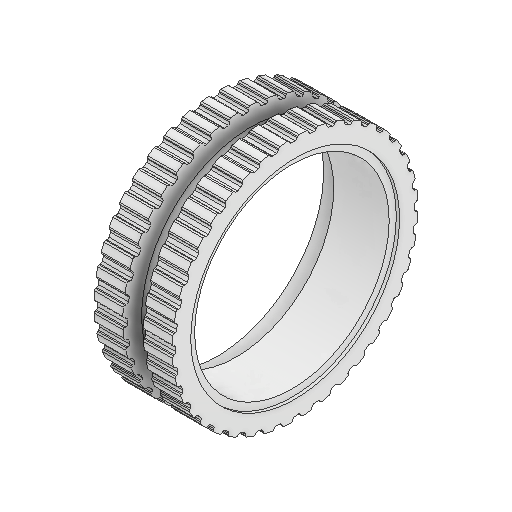
# Autodesk Inventor part: hoverboardPulleyAdapter
Saved by Autodesk Inventor 2025 (Build 290162000, 162)
## iProperties
Created: 2024-06-22
Part Number: hoverboardPulleyAdapter
Material: ABS Plastic
Document SubType Name: Modeling
Designer: derm
Density: 1.06 g/cm^3
Appearance: Smooth - White
Mass: 267.013 g
Surface Area: 496.078 cm^2
Volume: 251.899 cm^3
Author: derm
Autodesk Inventor part; units mm, degrees
ref_plane "YZ Plane" through (0, 0, 0) normal (1, 0, 0) x (0, 1, 0)
ref_plane "XZ Plane" through (0, 0, 0) normal (0, 1, 0) x (-1, 0, 0)
ref_plane "XY Plane" through (0, 0, 0) normal (0, 0, 1) x (1, 0, 0)
sketch "Sketch1" plane through (0, 0, 0) normal (1, 0, 0) x (0, 1, 0)
  circle A0 centre (0, 0) radius 63.119
  circle A1 centre (0, 0) radius 72.4459 projected
  arc A2 (-69.867, -16.1918) -> (-68.6025, -20.911) centre (0, 0) ccw projected
  arc A3 (-69.3853, -15.0825) -> (-69.867, -16.1918) centre (-68.8773, -15.9624) ccw projected
  line L0 (-69.3853, -15.0825) -> (-68.7891, -14.7383) projected
  arc A4 (-68.7891, -14.7383) -> (-68.0995, -13.2595) centre (-69.5003, -13.5065) ccw projected
  line L1 (-68.0995, -13.2595) -> (-68.5276, -10.8316) projected
  arc A5 (-68.5276, -10.8316) -> (-69.6814, -9.6778) centre (-69.9284, -11.0786) ccw projected
  line L2 (-69.6814, -9.6778) -> (-70.3594, -9.5582) projected
  arc A6 (-71.1915, -8.6806) -> (-70.3594, -9.5582) centre (-70.1829, -8.5577) ccw projected
  arc A7 (-71.6173, -3.8135) -> (-71.1915, -8.6806) centre (0, 0) ccw projected
  arc A8 (-70.9502, -2.8048) -> (-71.6173, -3.8135) centre (-70.6027, -3.7595) ccw projected
  line L3 (-70.9502, -2.8048) -> (-70.3033, -2.5693) projected
  arc A9 (-70.3033, -2.5693) -> (-69.3674, -1.2327) centre (-70.7898, -1.2327) ccw projected
  line L4 (-69.3674, -1.2327) -> (-69.3674, 1.2327) projected
  arc A10 (-69.3674, 1.2327) -> (-70.3033, 2.5693) centre (-70.7898, 1.2327) ccw projected
  line L5 (-70.3033, 2.5693) -> (-70.9502, 2.8048) projected
  arc A11 (-71.6173, 3.8135) -> (-70.9502, 2.8048) centre (-70.6027, 3.7595) ccw projected
  arc A12 (-71.1915, 8.6806) -> (-71.6173, 3.8135) centre (0, 0) ccw projected
  arc A13 (-70.3594, 9.5582) -> (-71.1915, 8.6806) centre (-70.1829, 8.5577) ccw projected
  line L6 (-70.3594, 9.5582) -> (-69.6814, 9.6778) projected
  arc A14 (-69.6814, 9.6778) -> (-68.5276, 10.8316) centre (-69.9284, 11.0786) ccw projected
  line L7 (-68.5276, 10.8316) -> (-68.0995, 13.2595) projected
  arc A15 (-68.0995, 13.2595) -> (-68.7891, 14.7383) centre (-69.5003, 13.5065) ccw projected
  line L8 (-68.7891, 14.7383) -> (-69.3853, 15.0825) projected
  arc A16 (-69.867, 16.1918) -> (-69.3853, 15.0825) centre (-68.8773, 15.9624) ccw projected
  arc A17 (-68.6025, 20.911) -> (-69.867, 16.1918) centre (0, 0) ccw projected
  arc A18 (-67.6307, 21.6308) -> (-68.6025, 20.911) centre (-67.6307, 20.6148) ccw projected
  line L9 (-67.6307, 21.6308) -> (-66.9423, 21.6308) projected
  arc A19 (-66.9423, 21.6308) -> (-65.6056, 22.5667) centre (-66.9423, 23.0532) ccw projected
  line L10 (-65.6056, 22.5667) -> (-64.7624, 24.8834) projected
  arc A20 (-64.7624, 24.8834) -> (-65.1847, 26.4595) centre (-66.099, 25.3699) ccw projected
  line L11 (-65.1847, 26.4595) -> (-65.7121, 26.902) projected
  arc A21 (-65.9939, 28.0781) -> (-65.7121, 26.902) centre (-65.059, 27.6803) ccw projected
  arc A22 (-63.9291, 32.506) -> (-65.9939, 28.0781) centre (0, 0) ccw projected
  arc A23 (-62.8471, 33.0461) -> (-63.9291, 32.506) centre (-63.0235, 32.0455) ccw projected
  line L12 (-62.8471, 33.0461) -> (-62.1691, 32.9266) projected
  arc A24 (-62.1691, 32.9266) -> (-60.6903, 33.6162) centre (-61.9221, 34.3274) ccw projected
  line L13 (-60.6903, 33.6162) -> (-59.4576, 35.7512) projected
  arc A25 (-59.4576, 35.7512) -> (-59.5998, 37.3767) centre (-60.6894, 36.4624) ccw projected
  line L14 (-59.5998, 37.3767) -> (-60.0423, 37.9041) projected
  arc A26 (-60.1156, 39.1112) -> (-60.0423, 37.9041) centre (-59.264, 38.5572) ccw projected
  arc A27 (-57.3133, 43.1134) -> (-60.1156, 39.1112) centre (0, 0) ccw projected
  arc A28 (-56.1539, 43.4573) -> (-57.3133, 43.1134) centre (-56.5014, 42.5026) ccw projected
  line L15 (-56.1539, 43.4573) -> (-55.507, 43.2219) projected
  arc A29 (-55.507, 43.2219) -> (-53.9309, 43.6442) centre (-55.0205, 44.5585) ccw projected
  line L16 (-53.9309, 43.6442) -> (-52.3462, 45.5328) projected
  arc A30 (-52.3462, 45.5328) -> (-52.2039, 47.1583) centre (-53.4358, 46.4471) ccw projected
  line L17 (-52.2039, 47.1583) -> (-52.5481, 47.7545) projected
  arc A31 (-52.4107, 48.956) -> (-52.5481, 47.7545) centre (-51.6683, 48.2625) ccw projected
  arc A32 (-48.956, 52.4107) -> (-52.4107, 48.956) centre (0, 0) ccw projected
  arc A33 (-47.7545, 52.5481) -> (-48.956, 52.4107) centre (-48.2625, 51.6683) ccw projected
  line L18 (-47.7545, 52.5481) -> (-47.1583, 52.2039) projected
  arc A34 (-47.1583, 52.2039) -> (-45.5328, 52.3462) centre (-46.4471, 53.4358) ccw projected
  line L19 (-45.5328, 52.3462) -> (-43.6442, 53.9309) projected
  arc A35 (-43.6442, 53.9309) -> (-43.2219, 55.507) centre (-44.5585, 55.0205) ccw projected
  line L20 (-43.2219, 55.507) -> (-43.4573, 56.1539) projected
  arc A36 (-43.1134, 57.3133) -> (-43.4573, 56.1539) centre (-42.5026, 56.5014) ccw projected
  arc A37 (-39.1112, 60.1156) -> (-43.1134, 57.3133) centre (0, 0) ccw projected
  arc A38 (-37.9041, 60.0423) -> (-39.1112, 60.1156) centre (-38.5572, 59.264) ccw projected
  line L21 (-37.9041, 60.0423) -> (-37.3767, 59.5998) projected
  arc A39 (-37.3767, 59.5998) -> (-35.7512, 59.4576) centre (-36.4624, 60.6894) ccw projected
  line L22 (-35.7512, 59.4576) -> (-33.6162, 60.6903) projected
  arc A40 (-33.6162, 60.6903) -> (-32.9266, 62.1691) centre (-34.3274, 61.9221) ccw projected
  line L23 (-32.9266, 62.1691) -> (-33.0461, 62.8471) projected
  arc A41 (-32.506, 63.9291) -> (-33.0461, 62.8471) centre (-32.0455, 63.0235) ccw projected
  arc A42 (-28.0781, 65.9939) -> (-32.506, 63.9291) centre (0, 0) ccw projected
  arc A43 (-26.902, 65.7121) -> (-28.0781, 65.9939) centre (-27.6803, 65.059) ccw projected
  line L24 (-26.902, 65.7121) -> (-26.4595, 65.1847) projected
  arc A44 (-26.4595, 65.1847) -> (-24.8834, 64.7624) centre (-25.3699, 66.099) ccw projected
  line L25 (-24.8834, 64.7624) -> (-22.5667, 65.6056) projected
  arc A45 (-22.5667, 65.6056) -> (-21.6308, 66.9423) centre (-23.0532, 66.9423) ccw projected
  line L26 (-21.6308, 66.9423) -> (-21.6308, 67.6307) projected
  arc A46 (-20.911, 68.6025) -> (-21.6308, 67.6307) centre (-20.6148, 67.6307) ccw projected
  arc A47 (-16.1918, 69.867) -> (-20.911, 68.6025) centre (0, 0) ccw projected
  arc A48 (-15.0825, 69.3853) -> (-16.1918, 69.867) centre (-15.9624, 68.8773) ccw projected
  line L27 (-15.0825, 69.3853) -> (-14.7383, 68.7891) projected
  arc A49 (-14.7383, 68.7891) -> (-13.2595, 68.0995) centre (-13.5065, 69.5003) ccw projected
  line L28 (-13.2595, 68.0995) -> (-10.8316, 68.5276) projected
  arc A50 (-10.8316, 68.5276) -> (-9.6778, 69.6814) centre (-11.0786, 69.9284) ccw projected
  line L29 (-9.6778, 69.6814) -> (-9.5582, 70.3594) projected
  arc A51 (-8.6806, 71.1915) -> (-9.5582, 70.3594) centre (-8.5577, 70.1829) ccw projected
  arc A52 (-3.8135, 71.6173) -> (-8.6806, 71.1915) centre (0, 0) ccw projected
  arc A53 (-2.8048, 70.9502) -> (-3.8135, 71.6173) centre (-3.7595, 70.6027) ccw projected
  line L30 (-2.8048, 70.9502) -> (-2.5693, 70.3033) projected
  arc A54 (-2.5693, 70.3033) -> (-1.2327, 69.3674) centre (-1.2327, 70.7898) ccw projected
  line L31 (-1.2327, 69.3674) -> (1.2327, 69.3674) projected
  arc A55 (1.2327, 69.3674) -> (2.5693, 70.3033) centre (1.2327, 70.7898) ccw projected
  line L32 (2.5693, 70.3033) -> (2.8048, 70.9502) projected
  arc A56 (3.8135, 71.6173) -> (2.8048, 70.9502) centre (3.7595, 70.6027) ccw projected
  arc A57 (8.6806, 71.1915) -> (3.8135, 71.6173) centre (0, 0) ccw projected
  arc A58 (9.5582, 70.3594) -> (8.6806, 71.1915) centre (8.5577, 70.1829) ccw projected
  line L33 (9.5582, 70.3594) -> (9.6778, 69.6814) projected
  arc A59 (9.6778, 69.6814) -> (10.8316, 68.5276) centre (11.0786, 69.9284) ccw projected
  line L34 (10.8316, 68.5276) -> (13.2595, 68.0995) projected
  arc A60 (13.2595, 68.0995) -> (14.7383, 68.7891) centre (13.5065, 69.5003) ccw projected
  line L35 (14.7383, 68.7891) -> (15.0825, 69.3853) projected
  arc A61 (16.1918, 69.867) -> (15.0825, 69.3853) centre (15.9624, 68.8773) ccw projected
  arc A62 (20.911, 68.6025) -> (16.1918, 69.867) centre (0, 0) ccw projected
  arc A63 (21.6308, 67.6307) -> (20.911, 68.6025) centre (20.6148, 67.6307) ccw projected
  line L36 (21.6308, 67.6307) -> (21.6308, 66.9423) projected
  arc A64 (21.6308, 66.9423) -> (22.5667, 65.6056) centre (23.0532, 66.9423) ccw projected
  line L37 (22.5667, 65.6056) -> (24.8834, 64.7624) projected
  arc A65 (24.8834, 64.7624) -> (26.4595, 65.1847) centre (25.3699, 66.099) ccw projected
  line L38 (26.4595, 65.1847) -> (26.902, 65.7121) projected
  arc A66 (28.0781, 65.9939) -> (26.902, 65.7121) centre (27.6803, 65.059) ccw projected
  arc A67 (32.506, 63.9291) -> (28.0781, 65.9939) centre (0, 0) ccw projected
  arc A68 (33.0461, 62.8471) -> (32.506, 63.9291) centre (32.0455, 63.0235) ccw projected
  line L39 (33.0461, 62.8471) -> (32.9266, 62.1691) projected
  arc A69 (32.9266, 62.1691) -> (33.6162, 60.6903) centre (34.3274, 61.9221) ccw projected
  line L40 (33.6162, 60.6903) -> (35.7512, 59.4576) projected
  arc A70 (35.7512, 59.4576) -> (37.3767, 59.5998) centre (36.4624, 60.6894) ccw projected
  line L41 (37.3767, 59.5998) -> (37.9041, 60.0423) projected
  arc A71 (39.1112, 60.1156) -> (37.9041, 60.0423) centre (38.5572, 59.264) ccw projected
  arc A72 (43.1134, 57.3133) -> (39.1112, 60.1156) centre (0, 0) ccw projected
  arc A73 (43.4573, 56.1539) -> (43.1134, 57.3133) centre (42.5026, 56.5014) ccw projected
  line L42 (43.4573, 56.1539) -> (43.2219, 55.507) projected
  arc A74 (43.2219, 55.507) -> (43.6442, 53.9309) centre (44.5585, 55.0205) ccw projected
  line L43 (43.6442, 53.9309) -> (45.5328, 52.3462) projected
  arc A75 (45.5328, 52.3462) -> (47.1583, 52.2039) centre (46.4471, 53.4358) ccw projected
  line L44 (47.1583, 52.2039) -> (47.7545, 52.5481) projected
  arc A76 (48.956, 52.4107) -> (47.7545, 52.5481) centre (48.2625, 51.6683) ccw projected
  arc A77 (52.4107, 48.956) -> (48.956, 52.4107) centre (0, 0) ccw projected
  arc A78 (52.5481, 47.7545) -> (52.4107, 48.956) centre (51.6683, 48.2625) ccw projected
  line L45 (52.5481, 47.7545) -> (52.2039, 47.1583) projected
  arc A79 (52.2039, 47.1583) -> (52.3462, 45.5328) centre (53.4358, 46.4471) ccw projected
  line L46 (52.3462, 45.5328) -> (53.9309, 43.6442) projected
  arc A80 (53.9309, 43.6442) -> (55.507, 43.2219) centre (55.0205, 44.5585) ccw projected
  line L47 (55.507, 43.2219) -> (56.1539, 43.4573) projected
  arc A81 (57.3133, 43.1134) -> (56.1539, 43.4573) centre (56.5014, 42.5026) ccw projected
  arc A82 (60.1156, 39.1112) -> (57.3133, 43.1134) centre (0, 0) ccw projected
  arc A83 (60.0423, 37.9041) -> (60.1156, 39.1112) centre (59.264, 38.5572) ccw projected
  line L48 (60.0423, 37.9041) -> (59.5998, 37.3767) projected
  arc A84 (59.5998, 37.3767) -> (59.4576, 35.7512) centre (60.6894, 36.4624) ccw projected
  line L49 (59.4576, 35.7512) -> (60.6903, 33.6162) projected
  arc A85 (60.6903, 33.6162) -> (62.1691, 32.9266) centre (61.9221, 34.3274) ccw projected
  line L50 (62.1691, 32.9266) -> (62.8471, 33.0461) projected
  arc A86 (63.9291, 32.506) -> (62.8471, 33.0461) centre (63.0235, 32.0455) ccw projected
  arc A87 (65.9939, 28.0781) -> (63.9291, 32.506) centre (0, 0) ccw projected
  arc A88 (65.7121, 26.902) -> (65.9939, 28.0781) centre (65.059, 27.6803) ccw projected
  line L51 (65.7121, 26.902) -> (65.1847, 26.4595) projected
  arc A89 (65.1847, 26.4595) -> (64.7624, 24.8834) centre (66.099, 25.3699) ccw projected
  line L52 (64.7624, 24.8834) -> (65.6056, 22.5667) projected
  arc A90 (65.6056, 22.5667) -> (66.9423, 21.6308) centre (66.9423, 23.0532) ccw projected
  line L53 (66.9423, 21.6308) -> (67.6307, 21.6308) projected
  arc A91 (68.6025, 20.911) -> (67.6307, 21.6308) centre (67.6307, 20.6148) ccw projected
  arc A92 (69.867, 16.1918) -> (68.6025, 20.911) centre (0, 0) ccw projected
  arc A93 (69.3853, 15.0825) -> (69.867, 16.1918) centre (68.8773, 15.9624) ccw projected
  line L54 (69.3853, 15.0825) -> (68.7891, 14.7383) projected
  arc A94 (68.7891, 14.7383) -> (68.0995, 13.2595) centre (69.5003, 13.5065) ccw projected
  line L55 (68.0995, 13.2595) -> (68.5276, 10.8316) projected
  arc A95 (68.5276, 10.8316) -> (69.6814, 9.6778) centre (69.9284, 11.0786) ccw projected
  line L56 (69.6814, 9.6778) -> (70.3594, 9.5582) projected
  arc A96 (71.1915, 8.6806) -> (70.3594, 9.5582) centre (70.1829, 8.5577) ccw projected
  arc A97 (71.6173, 3.8135) -> (71.1915, 8.6806) centre (0, 0) ccw projected
  arc A98 (70.9502, 2.8048) -> (71.6173, 3.8135) centre (70.6027, 3.7595) ccw projected
  line L57 (70.9502, 2.8048) -> (70.3033, 2.5693) projected
  arc A99 (70.3033, 2.5693) -> (69.3674, 1.2327) centre (70.7898, 1.2327) ccw projected
  line L58 (69.3674, 1.2327) -> (69.3674, -1.2327) projected
  arc A100 (69.3674, -1.2327) -> (70.3033, -2.5693) centre (70.7898, -1.2327) ccw projected
  line L59 (70.3033, -2.5693) -> (70.9502, -2.8048) projected
  arc A101 (71.6173, -3.8135) -> (70.9502, -2.8048) centre (70.6027, -3.7595) ccw projected
  arc A102 (71.1915, -8.6806) -> (71.6173, -3.8135) centre (0, 0) ccw projected
  arc A103 (70.3594, -9.5582) -> (71.1915, -8.6806) centre (70.1829, -8.5577) ccw projected
  line L60 (70.3594, -9.5582) -> (69.6814, -9.6778) projected
  arc A104 (69.6814, -9.6778) -> (68.5276, -10.8316) centre (69.9284, -11.0786) ccw projected
  line L61 (68.5276, -10.8316) -> (68.0995, -13.2595) projected
  arc A105 (68.0995, -13.2595) -> (68.7891, -14.7383) centre (69.5003, -13.5065) ccw projected
  line L62 (68.7891, -14.7383) -> (69.3853, -15.0825) projected
  arc A106 (69.867, -16.1918) -> (69.3853, -15.0825) centre (68.8773, -15.9624) ccw projected
  arc A107 (68.6025, -20.911) -> (69.867, -16.1918) centre (0, 0) ccw projected
  arc A108 (67.6307, -21.6308) -> (68.6025, -20.911) centre (67.6307, -20.6148) ccw projected
  line L63 (67.6307, -21.6308) -> (66.9423, -21.6308) projected
  arc A109 (66.9423, -21.6308) -> (65.6056, -22.5667) centre (66.9423, -23.0532) ccw projected
  line L64 (65.6056, -22.5667) -> (64.7624, -24.8834) projected
  arc A110 (64.7624, -24.8834) -> (65.1847, -26.4595) centre (66.099, -25.3699) ccw projected
  line L65 (65.1847, -26.4595) -> (65.7121, -26.902) projected
  arc A111 (65.9939, -28.0781) -> (65.7121, -26.902) centre (65.059, -27.6803) ccw projected
  arc A112 (63.9291, -32.506) -> (65.9939, -28.0781) centre (0, 0) ccw projected
  arc A113 (62.8471, -33.0461) -> (63.9291, -32.506) centre (63.0235, -32.0455) ccw projected
  line L66 (62.8471, -33.0461) -> (62.1691, -32.9266) projected
  arc A114 (62.1691, -32.9266) -> (60.6903, -33.6162) centre (61.9221, -34.3274) ccw projected
  line L67 (60.6903, -33.6162) -> (59.4576, -35.7512) projected
  arc A115 (59.4576, -35.7512) -> (59.5998, -37.3767) centre (60.6894, -36.4624) ccw projected
  line L68 (59.5998, -37.3767) -> (60.0423, -37.9041) projected
  arc A116 (60.1156, -39.1112) -> (60.0423, -37.9041) centre (59.264, -38.5572) ccw projected
  arc A117 (57.3133, -43.1134) -> (60.1156, -39.1112) centre (0, 0) ccw projected
  arc A118 (56.1539, -43.4573) -> (57.3133, -43.1134) centre (56.5014, -42.5026) ccw projected
  line L69 (56.1539, -43.4573) -> (55.507, -43.2219) projected
  arc A119 (55.507, -43.2219) -> (53.9309, -43.6442) centre (55.0205, -44.5585) ccw projected
  line L70 (53.9309, -43.6442) -> (52.3462, -45.5328) projected
  arc A120 (52.3462, -45.5328) -> (52.2039, -47.1583) centre (53.4358, -46.4471) ccw projected
  line L71 (52.2039, -47.1583) -> (52.5481, -47.7545) projected
  arc A121 (52.4107, -48.956) -> (52.5481, -47.7545) centre (51.6683, -48.2625) ccw projected
  arc A122 (48.956, -52.4107) -> (52.4107, -48.956) centre (0, 0) ccw projected
  arc A123 (47.7545, -52.5481) -> (48.956, -52.4107) centre (48.2625, -51.6683) ccw projected
  line L72 (47.7545, -52.5481) -> (47.1583, -52.2039) projected
  arc A124 (47.1583, -52.2039) -> (45.5328, -52.3462) centre (46.4471, -53.4358) ccw projected
  line L73 (45.5328, -52.3462) -> (43.6442, -53.9309) projected
  arc A125 (43.6442, -53.9309) -> (43.2219, -55.507) centre (44.5585, -55.0205) ccw projected
  line L74 (43.2219, -55.507) -> (43.4573, -56.1539) projected
  arc A126 (43.1134, -57.3133) -> (43.4573, -56.1539) centre (42.5026, -56.5014) ccw projected
  arc A127 (39.1112, -60.1156) -> (43.1134, -57.3133) centre (0, 0) ccw projected
  arc A128 (37.9041, -60.0423) -> (39.1112, -60.1156) centre (38.5572, -59.264) ccw projected
  line L75 (37.9041, -60.0423) -> (37.3767, -59.5998) projected
  arc A129 (37.3767, -59.5998) -> (35.7512, -59.4576) centre (36.4624, -60.6894) ccw projected
  line L76 (35.7512, -59.4576) -> (33.6162, -60.6903) projected
  arc A130 (33.6162, -60.6903) -> (32.9266, -62.1691) centre (34.3274, -61.9221) ccw projected
  line L77 (32.9266, -62.1691) -> (33.0461, -62.8471) projected
  arc A131 (32.506, -63.9291) -> (33.0461, -62.8471) centre (32.0455, -63.0235) ccw projected
  arc A132 (28.0781, -65.9939) -> (32.506, -63.9291) centre (0, 0) ccw projected
  arc A133 (26.902, -65.7121) -> (28.0781, -65.9939) centre (27.6803, -65.059) ccw projected
  line L78 (26.902, -65.7121) -> (26.4595, -65.1847) projected
  arc A134 (26.4595, -65.1847) -> (24.8834, -64.7624) centre (25.3699, -66.099) ccw projected
  line L79 (24.8834, -64.7624) -> (22.5667, -65.6056) projected
  arc A135 (22.5667, -65.6056) -> (21.6308, -66.9423) centre (23.0532, -66.9423) ccw projected
  line L80 (21.6308, -66.9423) -> (21.6308, -67.6307) projected
  arc A136 (20.911, -68.6025) -> (21.6308, -67.6307) centre (20.6148, -67.6307) ccw projected
  arc A137 (16.1918, -69.867) -> (20.911, -68.6025) centre (0, 0) ccw projected
  arc A138 (15.0825, -69.3853) -> (16.1918, -69.867) centre (15.9624, -68.8773) ccw projected
  line L81 (15.0825, -69.3853) -> (14.7383, -68.7891) projected
  arc A139 (14.7383, -68.7891) -> (13.2595, -68.0995) centre (13.5065, -69.5003) ccw projected
  line L82 (13.2595, -68.0995) -> (10.8316, -68.5276) projected
  arc A140 (10.8316, -68.5276) -> (9.6778, -69.6814) centre (11.0786, -69.9284) ccw projected
  line L83 (9.6778, -69.6814) -> (9.5582, -70.3594) projected
  arc A141 (8.6806, -71.1915) -> (9.5582, -70.3594) centre (8.5577, -70.1829) ccw projected
  arc A142 (3.8135, -71.6173) -> (8.6806, -71.1915) centre (0, 0) ccw projected
  arc A143 (2.8048, -70.9502) -> (3.8135, -71.6173) centre (3.7595, -70.6027) ccw projected
  line L84 (2.8048, -70.9502) -> (2.5693, -70.3033) projected
  arc A144 (2.5693, -70.3033) -> (1.2327, -69.3674) centre (1.2327, -70.7898) ccw projected
  line L85 (1.2327, -69.3674) -> (-1.2327, -69.3674) projected
  arc A145 (-1.2327, -69.3674) -> (-2.5693, -70.3033) centre (-1.2327, -70.7898) ccw projected
  line L86 (-2.5693, -70.3033) -> (-2.8048, -70.9502) projected
  arc A146 (-3.8135, -71.6173) -> (-2.8048, -70.9502) centre (-3.7595, -70.6027) ccw projected
  arc A147 (-8.6806, -71.1915) -> (-3.8135, -71.6173) centre (0, 0) ccw projected
  arc A148 (-9.5582, -70.3594) -> (-8.6806, -71.1915) centre (-8.5577, -70.1829) ccw projected
  line L87 (-9.5582, -70.3594) -> (-9.6778, -69.6814) projected
  arc A149 (-9.6778, -69.6814) -> (-10.8316, -68.5276) centre (-11.0786, -69.9284) ccw projected
  line L88 (-10.8316, -68.5276) -> (-13.2595, -68.0995) projected
  arc A150 (-13.2595, -68.0995) -> (-14.7383, -68.7891) centre (-13.5065, -69.5003) ccw projected
  line L89 (-14.7383, -68.7891) -> (-15.0825, -69.3853) projected
  arc A151 (-16.1918, -69.867) -> (-15.0825, -69.3853) centre (-15.9624, -68.8773) ccw projected
  arc A152 (-20.911, -68.6025) -> (-16.1918, -69.867) centre (0, 0) ccw projected
  arc A153 (-21.6308, -67.6307) -> (-20.911, -68.6025) centre (-20.6148, -67.6307) ccw projected
  line L90 (-21.6308, -67.6307) -> (-21.6308, -66.9423) projected
  arc A154 (-21.6308, -66.9423) -> (-22.5667, -65.6056) centre (-23.0532, -66.9423) ccw projected
  line L91 (-22.5667, -65.6056) -> (-24.8834, -64.7624) projected
  arc A155 (-24.8834, -64.7624) -> (-26.4595, -65.1847) centre (-25.3699, -66.099) ccw projected
  line L92 (-26.4595, -65.1847) -> (-26.902, -65.7121) projected
  arc A156 (-28.0781, -65.9939) -> (-26.902, -65.7121) centre (-27.6803, -65.059) ccw projected
  arc A157 (-32.506, -63.9291) -> (-28.0781, -65.9939) centre (0, 0) ccw projected
  arc A158 (-33.0461, -62.8471) -> (-32.506, -63.9291) centre (-32.0455, -63.0235) ccw projected
  line L93 (-33.0461, -62.8471) -> (-32.9266, -62.1691) projected
  arc A159 (-32.9266, -62.1691) -> (-33.6162, -60.6903) centre (-34.3274, -61.9221) ccw projected
  line L94 (-33.6162, -60.6903) -> (-35.7512, -59.4576) projected
  arc A160 (-35.7512, -59.4576) -> (-37.3767, -59.5998) centre (-36.4624, -60.6894) ccw projected
  line L95 (-37.3767, -59.5998) -> (-37.9041, -60.0423) projected
  arc A161 (-39.1112, -60.1156) -> (-37.9041, -60.0423) centre (-38.5572, -59.264) ccw projected
  arc A162 (-43.1134, -57.3133) -> (-39.1112, -60.1156) centre (0, 0) ccw projected
  arc A163 (-43.4573, -56.1539) -> (-43.1134, -57.3133) centre (-42.5026, -56.5014) ccw projected
  line L96 (-43.4573, -56.1539) -> (-43.2219, -55.507) projected
  arc A164 (-43.2219, -55.507) -> (-43.6442, -53.9309) centre (-44.5585, -55.0205) ccw projected
  line L97 (-43.6442, -53.9309) -> (-45.5328, -52.3462) projected
  arc A165 (-45.5328, -52.3462) -> (-47.1583, -52.2039) centre (-46.4471, -53.4358) ccw projected
  line L98 (-47.1583, -52.2039) -> (-47.7545, -52.5481) projected
  arc A166 (-48.956, -52.4107) -> (-47.7545, -52.5481) centre (-48.2625, -51.6683) ccw projected
  arc A167 (-52.4107, -48.956) -> (-48.956, -52.4107) centre (0, 0) ccw projected
  arc A168 (-52.5481, -47.7545) -> (-52.4107, -48.956) centre (-51.6683, -48.2625) ccw projected
  line L99 (-52.5481, -47.7545) -> (-52.2039, -47.1583) projected
  arc A169 (-52.2039, -47.1583) -> (-52.3462, -45.5328) centre (-53.4358, -46.4471) ccw projected
  line L100 (-52.3462, -45.5328) -> (-53.9309, -43.6442) projected
  arc A170 (-53.9309, -43.6442) -> (-55.507, -43.2219) centre (-55.0205, -44.5585) ccw projected
  line L101 (-55.507, -43.2219) -> (-56.1539, -43.4573) projected
  arc A171 (-57.3133, -43.1134) -> (-56.1539, -43.4573) centre (-56.5014, -42.5026) ccw projected
  arc A172 (-60.1156, -39.1112) -> (-57.3133, -43.1134) centre (0, 0) ccw projected
  arc A173 (-60.0423, -37.9041) -> (-60.1156, -39.1112) centre (-59.264, -38.5572) ccw projected
  line L102 (-60.0423, -37.9041) -> (-59.5998, -37.3767) projected
  arc A174 (-59.5998, -37.3767) -> (-59.4576, -35.7512) centre (-60.6894, -36.4624) ccw projected
  line L103 (-59.4576, -35.7512) -> (-60.6903, -33.6162) projected
  arc A175 (-60.6903, -33.6162) -> (-62.1691, -32.9266) centre (-61.9221, -34.3274) ccw projected
  line L104 (-62.1691, -32.9266) -> (-62.8471, -33.0461) projected
  arc A176 (-63.9291, -32.506) -> (-62.8471, -33.0461) centre (-63.0235, -32.0455) ccw projected
  arc A177 (-65.9939, -28.0781) -> (-63.9291, -32.506) centre (0, 0) ccw projected
  arc A178 (-65.7121, -26.902) -> (-65.9939, -28.0781) centre (-65.059, -27.6803) ccw projected
  line L105 (-65.7121, -26.902) -> (-65.1847, -26.4595) projected
  arc A179 (-65.1847, -26.4595) -> (-64.7624, -24.8834) centre (-66.099, -25.3699) ccw projected
  line L106 (-64.7624, -24.8834) -> (-65.6056, -22.5667) projected
  arc A180 (-65.6056, -22.5667) -> (-66.9423, -21.6308) centre (-66.9423, -23.0532) ccw projected
  line L107 (-66.9423, -21.6308) -> (-67.6307, -21.6308) projected
  arc A181 (-68.6025, -20.911) -> (-67.6307, -21.6308) centre (-67.6307, -20.6148) ccw projected
  circle A182 centre (0, 0) radius 80.5866 projected
  arc A183 (5.034, -79.6304) -> (9.9234, -79.1698) centre (0, 0) ccw projected
  arc A184 (9.9234, -79.1698) -> (10.7972, -78.3402) centre (9.797, -78.1617) ccw projected
  line L108 (10.7972, -78.3402) -> (10.9188, -77.6588) projected
  arc A185 (12.075, -76.5074) -> (10.9188, -77.6588) centre (12.3191, -77.9087) ccw projected
  line L109 (12.075, -76.5074) -> (14.5038, -76.0843) projected
  arc A186 (15.9812, -76.777) -> (14.5038, -76.0843) centre (14.7479, -77.4856) ccw projected
  line L110 (15.9812, -76.777) -> (16.3261, -77.3772) projected
  arc A187 (16.3261, -77.3772) -> (17.429, -77.8625) centre (17.207, -76.871) ccw projected
  arc A188 (17.429, -77.8625) -> (22.1861, -76.6428) centre (0, 0) ccw projected
  arc A189 (22.1861, -76.6428) -> (22.9194, -75.6867) centre (21.9036, -75.6668) ccw projected
  line L111 (22.9194, -75.6867) -> (22.9329, -74.9946) projected
  arc A190 (23.8947, -73.6765) -> (22.9329, -74.9946) centre (24.355, -75.0224) ccw projected
  line L112 (23.8947, -73.6765) -> (26.2275, -72.8787) projected
  arc A191 (27.795, -73.3317) -> (26.2275, -72.8787) centre (26.6878, -74.2246) ccw projected
  line L113 (27.795, -73.3317) -> (28.2295, -73.8706) projected
  arc A192 (28.2295, -73.8706) -> (29.3948, -74.1774) centre (29.0205, -73.2328) ccw projected
  arc A193 (29.3948, -74.1774) -> (33.9025, -72.2285) centre (0, 0) ccw projected
  arc A194 (33.9025, -72.2285) -> (34.4772, -71.1695) centre (33.4708, -71.3088) ccw projected
  line L114 (34.4772, -71.1695) -> (34.3823, -70.4838) projected
  arc A195 (35.1261, -69.0315) -> (34.3823, -70.4838) centre (35.7913, -70.2888) ccw projected
  line L115 (35.1261, -69.0315) -> (37.3053, -67.8786) projected
  arc A196 (38.9244, -68.0808) -> (37.3053, -67.8786) centre (37.9705, -69.1359) ccw projected
  line L116 (38.9244, -68.0808) -> (39.4379, -68.5451) projected
  arc A197 (39.4379, -68.5451) -> (40.6368, -68.6658) centre (40.1193, -67.7914) ccw projected
  arc A198 (40.6368, -68.6658) -> (44.7841, -66.0357) centre (0, 0) ccw projected
  arc A199 (44.7841, -66.0357) -> (45.1861, -64.8998) centre (44.2139, -65.1949) ccw projected
  line L117 (45.1861, -64.8998) -> (44.9851, -64.2374) projected
  arc A200 (45.4925, -62.6866) -> (44.9851, -64.2374) centre (46.3462, -63.8244) ccw projected
  line L118 (45.4925, -62.6866) -> (47.4646, -61.207) projected
  arc A201 (49.0954, -61.1535) -> (47.4646, -61.207) centre (48.3182, -62.3448) ccw projected
  line L119 (49.0954, -61.1535) -> (49.6752, -61.5317) projected
  arc A202 (49.6752, -61.5317) -> (50.8781, -61.4634) centre (50.2303, -60.6808) ccw projected
  arc A203 (50.8781, -61.4634) -> (54.563, -58.2169) centre (0, 0) ccw projected
  arc A204 (54.563, -58.2169) -> (54.7824, -57.0321) centre (53.8683, -57.4756) ccw projected
  line L120 (54.7824, -57.0321) -> (54.4802, -56.4093) projected
  arc A205 (54.7388, -54.7983) -> (54.4802, -56.4093) centre (55.7599, -55.7885) ccw projected
  line L121 (54.7388, -54.7983) -> (56.4551, -53.0284) projected
  arc A206 (58.0575, -52.7204) -> (56.4551, -53.0284) centre (57.4762, -54.0186) ccw projected
  line L122 (58.0575, -52.7204) -> (58.6893, -53.0032) projected
  arc A207 (58.6893, -53.0032) -> (59.8667, -52.7476) centre (59.1044, -52.0759) ccw projected
  arc A208 (59.8667, -52.7476) -> (62.9984, -48.9647) centre (0, 0) ccw projected
  arc A209 (62.9984, -48.9647) -> (63.0297, -47.7601) centre (62.1962, -48.3412) ccw projected
  line L123 (63.0297, -47.7601) -> (62.6338, -47.1923) projected
  arc A210 (62.6372, -45.5606) -> (62.6338, -47.1923) centre (63.8007, -46.3788) ccw projected
  line L124 (62.6372, -45.5606) -> (64.0555, -43.544) projected
  arc A211 (65.59, -42.9891) -> (64.0555, -43.544) centre (65.219, -44.3623) ccw projected
  line L125 (65.59, -42.9891) -> (66.2582, -43.1697) projected
  arc A212 (66.2582, -43.1697) -> (67.3812, -42.733) centre (66.5232, -42.1888) ccw projected
  arc A213 (67.3812, -42.733) -> (69.8826, -38.5067) centre (0, 0) ccw projected
  arc A214 (69.8826, -38.5067) -> (69.725, -37.3121) centre (68.9927, -38.0164) ccw projected
  line L126 (69.725, -37.3121) -> (69.2452, -36.8132) projected
  arc A215 (68.9933, -35.201) -> (69.2452, -36.8132) centre (70.2704, -35.8272) ccw projected
  line L127 (68.9933, -35.201) -> (70.0786, -32.9874) projected
  arc A216 (71.5074, -32.1993) -> (70.0786, -32.9874) centre (71.3558, -33.6136) ccw projected
  line L128 (71.5074, -32.1993) -> (72.1957, -32.2731) projected
  arc A217 (72.1957, -32.2731) -> (73.2366, -31.6661) centre (72.304, -31.2629) ccw projected
  arc A218 (73.2366, -31.6661) -> (75.046, -27.1006) centre (0, 0) ccw projected
  arc A219 (75.046, -27.1006) -> (74.7035, -25.9453) centre (74.0904, -26.7555) ccw projected
  line L129 (74.7035, -25.9453) -> (74.1515, -25.5276) projected
  arc A220 (73.6505, -23.9747) -> (74.1515, -25.5276) centre (75.0099, -24.3934) ccw projected
  line L130 (73.6505, -23.9747) -> (74.3762, -21.6186) projected
  arc A221 (75.6641, -20.6167) -> (74.3762, -21.6186) centre (75.7356, -22.0373) ccw projected
  line L131 (75.6641, -20.6167) -> (76.3555, -20.5819) projected
  arc A222 (76.3555, -20.5819) -> (77.2886, -19.8195) centre (76.3044, -19.5671) ccw projected
  arc A223 (77.2886, -19.8195) -> (78.3615, -15.0271) centre (0, 0) ccw projected
  arc A224 (78.3615, -15.0271) -> (77.8425, -13.9397) centre (77.3637, -14.8358) ccw projected
  line L132 (77.8425, -13.9397) -> (77.232, -13.6135) projected
  arc A225 (76.4942, -12.1581) -> (77.232, -13.6135) centre (77.9024, -12.3589) ccw projected
  line L133 (76.4942, -12.1581) -> (76.8424, -9.7174) projected
  arc A226 (77.9577, -8.5264) -> (76.8424, -9.7174) centre (78.2506, -9.9183) ccw projected
  line L134 (77.9577, -8.5264) -> (78.6351, -8.3838) projected
  arc A227 (78.6351, -8.3838) -> (79.4375, -7.4849) centre (78.426, -7.3896) ccw projected
  arc A228 (79.4375, -7.4849) -> (79.7475, -2.5837) centre (0, 0) ccw projected
  arc A229 (79.7475, -2.5837) -> (79.0648, -1.5908) centre (78.732, -2.5508) ccw projected
  line L135 (79.0648, -1.5908) -> (78.4107, -1.3641) projected
  arc A230 (77.4544, -0.042) -> (78.4107, -1.3641) centre (78.8766, -0.0202) ccw projected
  line L136 (77.4544, -0.042) -> (77.4165, 2.423) projected
  arc A231 (78.3318, 3.7739) -> (77.4165, 2.423) centre (78.8387, 2.4449) ccw projected
  line L137 (78.3318, 3.7739) -> (78.9785, 4.0206) projected
  arc A232 (78.9785, 4.0206) -> (79.6304, 5.034) centre (78.6164, 4.9699) ccw projected
  arc A233 (79.6304, 5.034) -> (79.1698, 9.9234) centre (0, 0) ccw projected
  arc A234 (79.1698, 9.9234) -> (78.3402, 10.7972) centre (78.1617, 9.797) ccw projected
  line L138 (78.3402, 10.7972) -> (77.6588, 10.9188) projected
  arc A235 (76.5074, 12.075) -> (77.6588, 10.9188) centre (77.9087, 12.3191) ccw projected
  line L139 (76.5074, 12.075) -> (76.0843, 14.5038) projected
  arc A236 (76.777, 15.9812) -> (76.0843, 14.5038) centre (77.4856, 14.7479) ccw projected
  line L140 (76.777, 15.9812) -> (77.3772, 16.3261) projected
  arc A237 (77.3772, 16.3261) -> (77.8625, 17.429) centre (76.871, 17.207) ccw projected
  arc A238 (77.8625, 17.429) -> (76.6428, 22.1861) centre (0, 0) ccw projected
  arc A239 (76.6428, 22.1861) -> (75.6867, 22.9194) centre (75.6668, 21.9036) ccw projected
  line L141 (75.6867, 22.9194) -> (74.9946, 22.9329) projected
  arc A240 (73.6765, 23.8947) -> (74.9946, 22.9329) centre (75.0224, 24.355) ccw projected
  line L142 (73.6765, 23.8947) -> (72.8787, 26.2275) projected
  arc A241 (73.3317, 27.795) -> (72.8787, 26.2275) centre (74.2246, 26.6878) ccw projected
  line L143 (73.3317, 27.795) -> (73.8706, 28.2295) projected
  arc A242 (73.8706, 28.2295) -> (74.1774, 29.3948) centre (73.2328, 29.0205) ccw projected
  arc A243 (74.1774, 29.3948) -> (72.2285, 33.9025) centre (0, 0) ccw projected
  arc A244 (72.2285, 33.9025) -> (71.1695, 34.4772) centre (71.3088, 33.4708) ccw projected
  line L144 (71.1695, 34.4772) -> (70.4838, 34.3823) projected
  arc A245 (69.0315, 35.1261) -> (70.4838, 34.3823) centre (70.2888, 35.7913) ccw projected
  line L145 (69.0315, 35.1261) -> (67.8786, 37.3053) projected
  arc A246 (68.0808, 38.9244) -> (67.8786, 37.3053) centre (69.1359, 37.9705) ccw projected
  line L146 (68.0808, 38.9244) -> (68.5451, 39.4379) projected
  arc A247 (68.5451, 39.4379) -> (68.6658, 40.6368) centre (67.7914, 40.1193) ccw projected
  arc A248 (68.6658, 40.6368) -> (66.0357, 44.7841) centre (0, 0) ccw projected
  arc A249 (66.0357, 44.7841) -> (64.8998, 45.1861) centre (65.1949, 44.2139) ccw projected
  line L147 (64.8998, 45.1861) -> (64.2374, 44.9851) projected
  arc A250 (62.6866, 45.4925) -> (64.2374, 44.9851) centre (63.8244, 46.3462) ccw projected
  line L148 (62.6866, 45.4925) -> (61.207, 47.4646) projected
  arc A251 (61.1535, 49.0954) -> (61.207, 47.4646) centre (62.3448, 48.3182) ccw projected
  line L149 (61.1535, 49.0954) -> (61.5317, 49.6752) projected
  arc A252 (61.5317, 49.6752) -> (61.4634, 50.8781) centre (60.6808, 50.2303) ccw projected
  arc A253 (61.4634, 50.8781) -> (58.2169, 54.563) centre (0, 0) ccw projected
  arc A254 (58.2169, 54.563) -> (57.0321, 54.7824) centre (57.4756, 53.8683) ccw projected
  line L150 (57.0321, 54.7824) -> (56.4093, 54.4802) projected
  arc A255 (54.7983, 54.7388) -> (56.4093, 54.4802) centre (55.7885, 55.7599) ccw projected
  line L151 (54.7983, 54.7388) -> (53.0284, 56.4551) projected
  arc A256 (52.7204, 58.0575) -> (53.0284, 56.4551) centre (54.0186, 57.4762) ccw projected
  line L152 (52.7204, 58.0575) -> (53.0032, 58.6893) projected
  arc A257 (53.0032, 58.6893) -> (52.7476, 59.8667) centre (52.0759, 59.1044) ccw projected
  arc A258 (52.7476, 59.8667) -> (48.9647, 62.9984) centre (0, 0) ccw projected
  arc A259 (48.9647, 62.9984) -> (47.7601, 63.0297) centre (48.3412, 62.1962) ccw projected
  line L153 (47.7601, 63.0297) -> (47.1923, 62.6338) projected
  arc A260 (45.5606, 62.6372) -> (47.1923, 62.6338) centre (46.3788, 63.8007) ccw projected
  line L154 (45.5606, 62.6372) -> (43.544, 64.0555) projected
  arc A261 (42.9891, 65.59) -> (43.544, 64.0555) centre (44.3623, 65.219) ccw projected
  line L155 (42.9891, 65.59) -> (43.1697, 66.2582) projected
  arc A262 (43.1697, 66.2582) -> (42.733, 67.3812) centre (42.1888, 66.5232) ccw projected
  arc A263 (42.733, 67.3812) -> (38.5067, 69.8826) centre (0, 0) ccw projected
  arc A264 (38.5067, 69.8826) -> (37.3121, 69.725) centre (38.0164, 68.9927) ccw projected
  line L156 (37.3121, 69.725) -> (36.8132, 69.2452) projected
  arc A265 (35.201, 68.9933) -> (36.8132, 69.2452) centre (35.8272, 70.2704) ccw projected
  line L157 (35.201, 68.9933) -> (32.9874, 70.0786) projected
  arc A266 (32.1993, 71.5074) -> (32.9874, 70.0786) centre (33.6136, 71.3558) ccw projected
  line L158 (32.1993, 71.5074) -> (32.2731, 72.1957) projected
  arc A267 (32.2731, 72.1957) -> (31.6661, 73.2366) centre (31.2629, 72.304) ccw projected
  arc A268 (31.6661, 73.2366) -> (27.1006, 75.046) centre (0, 0) ccw projected
  arc A269 (27.1006, 75.046) -> (25.9453, 74.7035) centre (26.7555, 74.0904) ccw projected
  line L159 (25.9453, 74.7035) -> (25.5276, 74.1515) projected
  arc A270 (23.9747, 73.6505) -> (25.5276, 74.1515) centre (24.3934, 75.0099) ccw projected
  line L160 (23.9747, 73.6505) -> (21.6186, 74.3762) projected
  arc A271 (20.6167, 75.6641) -> (21.6186, 74.3762) centre (22.0373, 75.7356) ccw projected
  line L161 (20.6167, 75.6641) -> (20.5819, 76.3555) projected
  arc A272 (20.5819, 76.3555) -> (19.8195, 77.2886) centre (19.5671, 76.3044) ccw projected
  arc A273 (19.8195, 77.2886) -> (15.0271, 78.3615) centre (0, 0) ccw projected
  arc A274 (15.0271, 78.3615) -> (13.9397, 77.8425) centre (14.8358, 77.3637) ccw projected
  line L162 (13.9397, 77.8425) -> (13.6135, 77.232) projected
  arc A275 (12.1581, 76.4942) -> (13.6135, 77.232) centre (12.3589, 77.9024) ccw projected
  line L163 (12.1581, 76.4942) -> (9.7174, 76.8424) projected
  arc A276 (8.5264, 77.9577) -> (9.7174, 76.8424) centre (9.9183, 78.2506) ccw projected
  line L164 (8.5264, 77.9577) -> (8.3838, 78.6351) projected
  arc A277 (8.3838, 78.6351) -> (7.4849, 79.4375) centre (7.3896, 78.426) ccw projected
  arc A278 (7.4849, 79.4375) -> (2.5837, 79.7475) centre (0, 0) ccw projected
  arc A279 (2.5837, 79.7475) -> (1.5908, 79.0648) centre (2.5508, 78.732) ccw projected
  line L165 (1.5908, 79.0648) -> (1.3641, 78.4107) projected
  arc A280 (0.042, 77.4544) -> (1.3641, 78.4107) centre (0.0202, 78.8766) ccw projected
  line L166 (0.042, 77.4544) -> (-2.423, 77.4165) projected
  arc A281 (-3.7739, 78.3318) -> (-2.423, 77.4165) centre (-2.4449, 78.8387) ccw projected
  line L167 (-3.7739, 78.3318) -> (-4.0206, 78.9785) projected
  arc A282 (-4.0206, 78.9785) -> (-5.034, 79.6304) centre (-4.9699, 78.6164) ccw projected
  arc A283 (-5.034, 79.6304) -> (-9.9234, 79.1698) centre (0, 0) ccw projected
  arc A284 (-9.9234, 79.1698) -> (-10.7972, 78.3402) centre (-9.797, 78.1617) ccw projected
  line L168 (-10.7972, 78.3402) -> (-10.9188, 77.6588) projected
  arc A285 (-12.075, 76.5074) -> (-10.9188, 77.6588) centre (-12.3191, 77.9087) ccw projected
  line L169 (-12.075, 76.5074) -> (-14.5038, 76.0843) projected
  arc A286 (-15.9812, 76.777) -> (-14.5038, 76.0843) centre (-14.7479, 77.4856) ccw projected
  line L170 (-15.9812, 76.777) -> (-16.3261, 77.3772) projected
  arc A287 (-16.3261, 77.3772) -> (-17.429, 77.8625) centre (-17.207, 76.871) ccw projected
  arc A288 (-17.429, 77.8625) -> (-22.1861, 76.6428) centre (0, 0) ccw projected
  arc A289 (-22.1861, 76.6428) -> (-22.9194, 75.6867) centre (-21.9036, 75.6668) ccw projected
  line L171 (-22.9194, 75.6867) -> (-22.9329, 74.9946) projected
  arc A290 (-23.8947, 73.6765) -> (-22.9329, 74.9946) centre (-24.355, 75.0224) ccw projected
  line L172 (-23.8947, 73.6765) -> (-26.2275, 72.8787) projected
  arc A291 (-27.795, 73.3317) -> (-26.2275, 72.8787) centre (-26.6878, 74.2246) ccw projected
  line L173 (-27.795, 73.3317) -> (-28.2295, 73.8706) projected
  arc A292 (-28.2295, 73.8706) -> (-29.3948, 74.1774) centre (-29.0205, 73.2328) ccw projected
  arc A293 (-29.3948, 74.1774) -> (-33.9025, 72.2285) centre (0, 0) ccw projected
  arc A294 (-33.9025, 72.2285) -> (-34.4772, 71.1695) centre (-33.4708, 71.3088) ccw projected
  line L174 (-34.4772, 71.1695) -> (-34.3823, 70.4838) projected
  arc A295 (-35.1261, 69.0315) -> (-34.3823, 70.4838) centre (-35.7913, 70.2888) ccw projected
  line L175 (-35.1261, 69.0315) -> (-37.3053, 67.8786) projected
  arc A296 (-38.9244, 68.0808) -> (-37.3053, 67.8786) centre (-37.9705, 69.1359) ccw projected
  line L176 (-38.9244, 68.0808) -> (-39.4379, 68.5451) projected
  arc A297 (-39.4379, 68.5451) -> (-40.6368, 68.6658) centre (-40.1193, 67.7914) ccw projected
  arc A298 (-40.6368, 68.6658) -> (-44.7841, 66.0357) centre (0, 0) ccw projected
  arc A299 (-44.7841, 66.0357) -> (-45.1861, 64.8998) centre (-44.2139, 65.1949) ccw projected
  line L177 (-45.1861, 64.8998) -> (-44.9851, 64.2374) projected
  arc A300 (-45.4925, 62.6866) -> (-44.9851, 64.2374) centre (-46.3462, 63.8244) ccw projected
  line L178 (-45.4925, 62.6866) -> (-47.4646, 61.207) projected
  arc A301 (-49.0954, 61.1535) -> (-47.4646, 61.207) centre (-48.3182, 62.3448) ccw projected
  line L179 (-49.0954, 61.1535) -> (-49.6752, 61.5317) projected
  arc A302 (-49.6752, 61.5317) -> (-50.8781, 61.4634) centre (-50.2303, 60.6808) ccw projected
  arc A303 (-50.8781, 61.4634) -> (-54.563, 58.2169) centre (0, 0) ccw projected
  arc A304 (-54.563, 58.2169) -> (-54.7824, 57.0321) centre (-53.8683, 57.4756) ccw projected
  line L180 (-54.7824, 57.0321) -> (-54.4802, 56.4093) projected
  arc A305 (-54.7388, 54.7983) -> (-54.4802, 56.4093) centre (-55.7599, 55.7885) ccw projected
  line L181 (-54.7388, 54.7983) -> (-56.4551, 53.0284) projected
  arc A306 (-58.0575, 52.7204) -> (-56.4551, 53.0284) centre (-57.4762, 54.0186) ccw projected
  line L182 (-58.0575, 52.7204) -> (-58.6893, 53.0032) projected
  arc A307 (-58.6893, 53.0032) -> (-59.8667, 52.7476) centre (-59.1044, 52.0759) ccw projected
  arc A308 (-59.8667, 52.7476) -> (-62.9984, 48.9647) centre (0, 0) ccw projected
  arc A309 (-62.9984, 48.9647) -> (-63.0297, 47.7601) centre (-62.1962, 48.3412) ccw projected
  line L183 (-63.0297, 47.7601) -> (-62.6338, 47.1923) projected
  arc A310 (-62.6372, 45.5606) -> (-62.6338, 47.1923) centre (-63.8007, 46.3788) ccw projected
  line L184 (-62.6372, 45.5606) -> (-64.0555, 43.544) projected
  arc A311 (-65.59, 42.9891) -> (-64.0555, 43.544) centre (-65.219, 44.3623) ccw projected
  line L185 (-65.59, 42.9891) -> (-66.2582, 43.1697) projected
  arc A312 (-66.2582, 43.1697) -> (-67.3812, 42.733) centre (-66.5232, 42.1888) ccw projected
  arc A313 (-67.3812, 42.733) -> (-69.8826, 38.5067) centre (0, 0) ccw projected
  arc A314 (-69.8826, 38.5067) -> (-69.725, 37.3121) centre (-68.9927, 38.0164) ccw projected
  line L186 (-69.725, 37.3121) -> (-69.2452, 36.8132) projected
  arc A315 (-68.9933, 35.201) -> (-69.2452, 36.8132) centre (-70.2704, 35.8272) ccw projected
  line L187 (-68.9933, 35.201) -> (-70.0786, 32.9874) projected
  arc A316 (-71.5074, 32.1993) -> (-70.0786, 32.9874) centre (-71.3558, 33.6136) ccw projected
  line L188 (-71.5074, 32.1993) -> (-72.1957, 32.2731) projected
  arc A317 (-72.1957, 32.2731) -> (-73.2366, 31.6661) centre (-72.304, 31.2629) ccw projected
  arc A318 (-73.2366, 31.6661) -> (-75.046, 27.1006) centre (0, 0) ccw projected
  arc A319 (-75.046, 27.1006) -> (-74.7035, 25.9453) centre (-74.0904, 26.7555) ccw projected
  line L189 (-74.7035, 25.9453) -> (-74.1515, 25.5276) projected
  arc A320 (-73.6505, 23.9747) -> (-74.1515, 25.5276) centre (-75.0099, 24.3934) ccw projected
  line L190 (-73.6505, 23.9747) -> (-74.3762, 21.6186) projected
  arc A321 (-75.6641, 20.6167) -> (-74.3762, 21.6186) centre (-75.7356, 22.0373) ccw projected
  line L191 (-75.6641, 20.6167) -> (-76.3555, 20.5819) projected
  arc A322 (-76.3555, 20.5819) -> (-77.2886, 19.8195) centre (-76.3044, 19.5671) ccw projected
  arc A323 (-77.2886, 19.8195) -> (-78.3615, 15.0271) centre (0, 0) ccw projected
  arc A324 (-78.3615, 15.0271) -> (-77.8425, 13.9397) centre (-77.3637, 14.8358) ccw projected
  line L192 (-77.8425, 13.9397) -> (-77.232, 13.6135) projected
  arc A325 (-76.4942, 12.1581) -> (-77.232, 13.6135) centre (-77.9024, 12.3589) ccw projected
  line L193 (-76.4942, 12.1581) -> (-76.8424, 9.7174) projected
  arc A326 (-77.9577, 8.5264) -> (-76.8424, 9.7174) centre (-78.2506, 9.9183) ccw projected
  line L194 (-77.9577, 8.5264) -> (-78.6351, 8.3838) projected
  arc A327 (-78.6351, 8.3838) -> (-79.4375, 7.4849) centre (-78.426, 7.3896) ccw projected
  arc A328 (-79.4375, 7.4849) -> (-79.7475, 2.5837) centre (0, 0) ccw projected
  arc A329 (-79.7475, 2.5837) -> (-79.0648, 1.5908) centre (-78.732, 2.5508) ccw projected
  line L195 (-79.0648, 1.5908) -> (-78.4107, 1.3641) projected
  arc A330 (-77.4544, 0.042) -> (-78.4107, 1.3641) centre (-78.8766, 0.0202) ccw projected
  line L196 (-77.4544, 0.042) -> (-77.4165, -2.423) projected
  arc A331 (-78.3318, -3.7739) -> (-77.4165, -2.423) centre (-78.8387, -2.4449) ccw projected
  line L197 (-78.3318, -3.7739) -> (-78.9785, -4.0206) projected
  arc A332 (-78.9785, -4.0206) -> (-79.6304, -5.034) centre (-78.6164, -4.9699) ccw projected
  arc A333 (-79.6304, -5.034) -> (-79.1698, -9.9234) centre (0, 0) ccw projected
  arc A334 (-79.1698, -9.9234) -> (-78.3402, -10.7972) centre (-78.1617, -9.797) ccw projected
  line L198 (-78.3402, -10.7972) -> (-77.6588, -10.9188) projected
  arc A335 (-76.5074, -12.075) -> (-77.6588, -10.9188) centre (-77.9087, -12.3191) ccw projected
  line L199 (-76.5074, -12.075) -> (-76.0843, -14.5038) projected
  arc A336 (-76.777, -15.9812) -> (-76.0843, -14.5038) centre (-77.4856, -14.7479) ccw projected
  line L200 (-76.777, -15.9812) -> (-77.3772, -16.3261) projected
  arc A337 (-77.3772, -16.3261) -> (-77.8625, -17.429) centre (-76.871, -17.207) ccw projected
  arc A338 (-77.8625, -17.429) -> (-76.6428, -22.1861) centre (0, 0) ccw projected
  arc A339 (-76.6428, -22.1861) -> (-75.6867, -22.9194) centre (-75.6668, -21.9036) ccw projected
  line L201 (-75.6867, -22.9194) -> (-74.9946, -22.9329) projected
  arc A340 (-73.6765, -23.8947) -> (-74.9946, -22.9329) centre (-75.0224, -24.355) ccw projected
  line L202 (-73.6765, -23.8947) -> (-72.8787, -26.2275) projected
  arc A341 (-73.3317, -27.795) -> (-72.8787, -26.2275) centre (-74.2246, -26.6878) ccw projected
  line L203 (-73.3317, -27.795) -> (-73.8706, -28.2295) projected
  arc A342 (-73.8706, -28.2295) -> (-74.1774, -29.3948) centre (-73.2328, -29.0205) ccw projected
  arc A343 (-74.1774, -29.3948) -> (-72.2285, -33.9025) centre (0, 0) ccw projected
  arc A344 (-72.2285, -33.9025) -> (-71.1695, -34.4772) centre (-71.3088, -33.4708) ccw projected
  line L204 (-71.1695, -34.4772) -> (-70.4838, -34.3823) projected
  arc A345 (-69.0315, -35.1261) -> (-70.4838, -34.3823) centre (-70.2888, -35.7913) ccw projected
  line L205 (-69.0315, -35.1261) -> (-67.8786, -37.3053) projected
  arc A346 (-68.0808, -38.9244) -> (-67.8786, -37.3053) centre (-69.1359, -37.9705) ccw projected
  line L206 (-68.0808, -38.9244) -> (-68.5451, -39.4379) projected
  arc A347 (-68.5451, -39.4379) -> (-68.6658, -40.6368) centre (-67.7914, -40.1193) ccw projected
  arc A348 (-68.6658, -40.6368) -> (-66.0357, -44.7841) centre (0, 0) ccw projected
  arc A349 (-66.0357, -44.7841) -> (-64.8998, -45.1861) centre (-65.1949, -44.2139) ccw projected
  line L207 (-64.8998, -45.1861) -> (-64.2374, -44.9851) projected
  arc A350 (-62.6866, -45.4925) -> (-64.2374, -44.9851) centre (-63.8244, -46.3462) ccw projected
  line L208 (-62.6866, -45.4925) -> (-61.207, -47.4646) projected
  arc A351 (-61.1535, -49.0954) -> (-61.207, -47.4646) centre (-62.3448, -48.3182) ccw projected
  line L209 (-61.1535, -49.0954) -> (-61.5317, -49.6752) projected
  arc A352 (-61.5317, -49.6752) -> (-61.4634, -50.8781) centre (-60.6808, -50.2303) ccw projected
  arc A353 (-61.4634, -50.8781) -> (-58.2169, -54.563) centre (0, 0) ccw projected
  arc A354 (-58.2169, -54.563) -> (-57.0321, -54.7824) centre (-57.4756, -53.8683) ccw projected
  line L210 (-57.0321, -54.7824) -> (-56.4093, -54.4802) projected
  arc A355 (-54.7983, -54.7388) -> (-56.4093, -54.4802) centre (-55.7885, -55.7599) ccw projected
  line L211 (-54.7983, -54.7388) -> (-53.0284, -56.4551) projected
  arc A356 (-52.7204, -58.0575) -> (-53.0284, -56.4551) centre (-54.0186, -57.4762) ccw projected
  line L212 (-52.7204, -58.0575) -> (-53.0032, -58.6893) projected
  arc A357 (-53.0032, -58.6893) -> (-52.7476, -59.8667) centre (-52.0759, -59.1044) ccw projected
  arc A358 (-52.7476, -59.8667) -> (-48.9647, -62.9984) centre (0, 0) ccw projected
  arc A359 (-48.9647, -62.9984) -> (-47.7601, -63.0297) centre (-48.3412, -62.1962) ccw projected
  line L213 (-47.7601, -63.0297) -> (-47.1923, -62.6338) projected
  arc A360 (-45.5606, -62.6372) -> (-47.1923, -62.6338) centre (-46.3788, -63.8007) ccw projected
  line L214 (-45.5606, -62.6372) -> (-43.544, -64.0555) projected
  arc A361 (-42.9891, -65.59) -> (-43.544, -64.0555) centre (-44.3623, -65.219) ccw projected
  line L215 (-42.9891, -65.59) -> (-43.1697, -66.2582) projected
  arc A362 (-43.1697, -66.2582) -> (-42.733, -67.3812) centre (-42.1888, -66.5232) ccw projected
  arc A363 (-42.733, -67.3812) -> (-38.5067, -69.8826) centre (0, 0) ccw projected
  arc A364 (-38.5067, -69.8826) -> (-37.3121, -69.725) centre (-38.0164, -68.9927) ccw projected
  line L216 (-37.3121, -69.725) -> (-36.8132, -69.2452) projected
  arc A365 (-35.201, -68.9933) -> (-36.8132, -69.2452) centre (-35.8272, -70.2704) ccw projected
  line L217 (-35.201, -68.9933) -> (-32.9874, -70.0786) projected
  arc A366 (-32.1993, -71.5074) -> (-32.9874, -70.0786) centre (-33.6136, -71.3558) ccw projected
  line L218 (-32.1993, -71.5074) -> (-32.2731, -72.1957) projected
  arc A367 (-32.2731, -72.1957) -> (-31.6661, -73.2366) centre (-31.2629, -72.304) ccw projected
  arc A368 (-31.6661, -73.2366) -> (-27.1006, -75.046) centre (0, 0) ccw projected
  arc A369 (-27.1006, -75.046) -> (-25.9453, -74.7035) centre (-26.7555, -74.0904) ccw projected
  line L219 (-25.9453, -74.7035) -> (-25.5276, -74.1515) projected
  arc A370 (-23.9747, -73.6505) -> (-25.5276, -74.1515) centre (-24.3934, -75.0099) ccw projected
  line L220 (-23.9747, -73.6505) -> (-21.6186, -74.3762) projected
  arc A371 (-20.6167, -75.6641) -> (-21.6186, -74.3762) centre (-22.0373, -75.7356) ccw projected
  line L221 (-20.6167, -75.6641) -> (-20.5819, -76.3555) projected
  arc A372 (-20.5819, -76.3555) -> (-19.8195, -77.2886) centre (-19.5671, -76.3044) ccw projected
  arc A373 (-19.8195, -77.2886) -> (-15.0271, -78.3615) centre (0, 0) ccw projected
  arc A374 (-15.0271, -78.3615) -> (-13.9397, -77.8425) centre (-14.8358, -77.3637) ccw projected
  line L222 (-13.9397, -77.8425) -> (-13.6135, -77.232) projected
  arc A375 (-12.1581, -76.4942) -> (-13.6135, -77.232) centre (-12.3589, -77.9024) ccw projected
  line L223 (-12.1581, -76.4942) -> (-9.7174, -76.8424) projected
  arc A376 (-8.5264, -77.9577) -> (-9.7174, -76.8424) centre (-9.9183, -78.2506) ccw projected
  line L224 (-8.5264, -77.9577) -> (-8.3838, -78.6351) projected
  arc A377 (-8.3838, -78.6351) -> (-7.4849, -79.4375) centre (-7.3896, -78.426) ccw projected
  arc A378 (-7.4849, -79.4375) -> (-2.5837, -79.7475) centre (0, 0) ccw projected
  arc A379 (-2.5837, -79.7475) -> (-1.5908, -79.0648) centre (-2.5508, -78.732) ccw projected
  line L225 (-1.5908, -79.0648) -> (-1.3641, -78.4107) projected
  arc A380 (-0.042, -77.4544) -> (-1.3641, -78.4107) centre (-0.0202, -78.8766) ccw projected
  line L226 (-0.042, -77.4544) -> (2.423, -77.4165) projected
  arc A381 (3.7739, -78.3318) -> (2.423, -77.4165) centre (2.4449, -78.8387) ccw projected
  line L227 (3.7739, -78.3318) -> (4.0206, -78.9785) projected
  arc A382 (4.0206, -78.9785) -> (5.034, -79.6304) centre (4.9699, -78.6164) ccw projected
  dimension "d0" = 126.238
  constraints: 1 centre point, 1 coincident
  measures "d0" diameter of A0
extrude "Extrusion1" add sketch "Sketch1" along normal mid plane 50.8 contours A1 | A3 L0 A4 L1 A5 L2 A6 A7 A8 L3 A9 L4 A10 L5 A11 A12 A13 L6 A14 L7 A15 L8 A16 A17 A18 L9 A19 L10 A20 L11 A21 A22 A23 L12 A24 L13 A25 L14 A26 A27 A28 L15 A29 L16 A30 L17 A31 A32 A33 L18 A34 L19 A35 L20 A36 A37 A38 L21 A39 L22 A40 L23 A41 A42 A43 L24 A44 L25 A45 L26 A46 A47 A48 L27 A49 L28 A50 L29 A51 A52 A53 L30 A54 L31 A55 L32 A56 A57 A58 L33 A59 L34 A60 L35 A61 A62 A63 L36 A64 L37 A65 L38 A66 A67 A68 L39 A69 L40 A70 L41 A71 A72 A73 L42 A74 L43 A75 L44 A76 A77 A78 L45 A79 L46 A80 L47 A81 A82 A83 L48 A84 L49 A85 L50 A86 A87 A88 L51 A89 L52 A90 L53 A91 A92 A93 L54 A94 L55 A95 L56 A96 A97 A98 L57 A99 L58 A100 L59 A101 A102 A103 L60 A104 L61 A105 L62 A106 A107 A108 L63 A109 L64 A110 L65 A111 A112 A113 L66 A114 L67 A115 L68 A116 A117 A118 L69 A119 L70 A120 L71 A121 A122 A123 L72 A124 L73 A125 L74 A126 A127 A128 L75 A129 L76 A130 L77 A131 A132 A133 L78 A134 L79 A135 L80 A136 A137 A138 L81 A139 L82 A140 L83 A141 A142 A143 L84 A144 L85 A145 L86 A146 A147 A148 L87 A149 L88 A150 L89 A151 A152 A153 L90 A154 L91 A155 L92 A156 A157 A158 L93 A159 L94 A160 L95 A161 A162 A163 L96 A164 L97 A165 L98 A166 A167 A168 L99 A169 L100 A170 L101 A171 A172 A173 L102 A174 L103 A175 L104 A176 A177 A178 L105 A179 L106 A180 L107 A181 A2 | A382 L227 A381 L226 A380 L225 A379 A378 A377 L224 A376 L223 A375 L222 A374 A373 A372 L221 A371 L220 A370 L219 A369 A368 A367 L218 A366 L217 A365 L216 A364 A363 A362 L215 A361 L214 A360 L213 A359 A358 A357 L212 A356 L211 A355 L210 A354 A353 A352 L209 A351 L208 A350 L207 A349 A348 A347 L206 A346 L205 A345 L204 A344 A343 A342 L203 A341 L202 A340 L201 A339 A338 A337 L200 A336 L199 A335 L198 A334 A333 A332 L197 A331 L196 A330 L195 A329 A328 A327 L194 A326 L193 A325 L192 A324 A323 A322 L191 A321 L190 A320 L189 A319 A318 A317 L188 A316 L187 A315 L186 A314 A313 A312 L185 A311 L184 A310 L183 A309 A308 A307 L182 A306 L181 A305 L180 A304 A303 A302 L179 A301 L178 A300 L177 A299 A298 A297 L176 A296 L175 A295 L174 A294 A293 A292 L173 A291 L172 A290 L171 A289 A288 A287 L170 A286 L169 A285 L168 A284 A283 A282 L167 A281 L166 A280 L165 A279 A278 A277 L164 A276 L163 A275 L162 A274 A273 A272 L161 A271 L160 A270 L159 A269 A268 A267 L158 A266 L157 A265 L156 A264 A263 A262 L155 A261 L154 A260 L153 A259 A258 A257 L152 A256 L151 A255 L150 A254 A253 A252 L149 A251 L148 A250 L147 A249 A248 A247 L146 A246 L145 A245 L144 A244 A243 A242 L143 A241 L142 A240 L141 A239 A238 A237 L140 A236 L139 A235 L138 A234 A233 A232 L137 A231 L136 A230 L135 A229 A228 A227 L134 A226 L133 A225 L132 A224 A223 A222 L131 A221 L130 A220 L129 A219 A218 A217 L128 A216 L127 A215 L126 A214 A213 A212 L125 A211 L124 A210 L123 A209 A208 A207 L122 A206 L121 A205 L120 A204 A203 A202 L119 A201 L118 A200 L117 A199 A198 A197 L116 A196 L115 A195 L114 A194 A193 A192 L113 A191 L112 A190 L111 A189 A188 A187 L110 A186 L109 A185 L108 A184 A183
sketch "Sketch2" plane through (0, 0, 0) normal (0, 1, 0) x (-1, 0, 0)
  line L0 (25.4, -79.7475) -> (-25.4, -79.7475) projected
  line L1 (0, -79.7475) -> (-6.6548, -79.7475)
  line L2 (0, -79.7475) -> (0, -70.8575)
  line L3 (0, -70.8575) -> (-3.3274, -70.8575)
  line L4 (25.4, -67.3812) -> (-25.4, -67.3812) projected
  line L5 (-3.3274, -70.8575) -> (-6.6548, -79.7475)
  line L6 (-6.6548, -79.7475) -> (-7.9914, -83.3185)
  line L7 (-7.9914, -83.3185) -> (0, -83.3185)
  line L8 (25.4, -79.0648) -> (-25.4, -79.0648) projected
  line L9 (0, -83.3185) -> (0, -79.7475)
  line L10 (0, 0) -> (56.0992, 0)
  dimension "d3" = 3.3274
  dimension "d4" = 6.6548
  dimension "d5" = 8.89
  constraints: 16 end point, 2 collinear, 2 parallel, 1 horizontal, 1 midpoint, 1 point on line, 1 vertical
  measures "d3" distance of L2.end L3.end
  measures "d4" distance from line of L1.end L2
  measures "d5" distance of L1.start L2.end
revolve "Revolution1" cut sketch "Sketch2" angle 360 about axis through (0, 0, 0) along (-1, 0, 0)
mirror "Mirror1" about plane through (0, 0, 0) normal (1, 0, 0) of "Revolution1"
sketch "Sketch3" plane through (-25.4, 0, 0) normal (-1, 0, 0) x (0, 0, 1)
  circle A0 centre (0, 0) radius 63.119 projected
  circle A1 centre (0, 0) radius 63.119 projected
  circle A2 centre (0, 0) radius 69.25
  dimension "d7" = 138.5
  constraints: 1 centre point, 1 coincident
  measures "d7" diameter of A2
extrude "Extrusion2" cut sketch "Sketch3" against normal blind 12.7
sketch "Sketch4" plane through (25.4, 0, 0) normal (1, 0, 0) x (0, 0, -1)
  circle A0 centre (0, 0) radius 63.119 projected
  circle A1 centre (0, 0) radius 67.75
  dimension "d10" = 135.5
  constraints: 1 centre point, 1 coincident
  measures "d10" diameter of A1
extrude "Extrusion3" cut sketch "Sketch4" against normal blind 2.1
body "Solid1"
